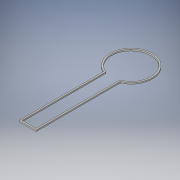
# Autodesk Inventor part: Arm Layer 2 Out
Saved by Autodesk Inventor 2016 (Build 200138000, 138)
## iProperties
Created: 2016-04-16
Part Number: Arm Layer 2 Out
Material: Generic
Document SubType Name: Modeling
Designer: rmarkowi
Density: 1 g/cm^3
Appearance: Default
Author: rmarkowi
Autodesk Inventor part; units mm, degrees
ref_plane "YZ Plane" through (0, 0, 0) normal (1, 0, 0) x (0, 1, 0)
ref_plane "XZ Plane" through (0, 0, 0) normal (0, 1, 0) x (-1, 0, 0)
ref_plane "XY Plane" through (0, 0, 0) normal (0, 0, 1) x (1, 0, 0)
sketch "Sketch1" plane through (0, 0, 0) normal (0, 1, 0) x (-1, 0, 0)
  line L0 (0, 0) -> (152.4, 0)
  line L1 (152.4, 0) -> (152.4, -762)
  line L2 (0, -762) -> (0, 0)
  line L3 (152.4, -762) -> (0, -762) construction
  arc A0 (0, -762) -> (152.4, -762) centre (76.2, -936.5961) ccw
  line L4 (152.4, -590.1365) -> (152.4, -762) construction
  arc A1 (12.7, -770.5221) -> (139.7, -770.5221) centre (76.2, -936.5961) ccw
  line L5 (12.7, -12.7) -> (139.7, -12.7)
  line L6 (139.7, -12.7) -> (139.7, -749.3)
  line L7 (12.7, -749.3) -> (12.7, -12.7)
  line L8 (12.7, -12.7) -> (139.7, -749.3) construction
  line L9 (139.7, -12.7) -> (12.7, -749.3) construction
  line L10 (12.7, -749.3) -> (12.7, -770.5221)
  line L11 (139.7, -749.3) -> (139.7, -770.5221)
  point P0 (76.2, -381)
  dimension "d0" = 762
  dimension "d1" = 381
  dimension "d2" = 355.6
  dimension "d3" = 762
  dimension "d4" = 127
  dimension "d5" = 736.6
  constraints: 24 end point, 4 point on circle, 3 parallel, 3 perpendicular, 2 centre point, 2 horizontal, 2 midpoint, 1 coincident, 1 collinear, 1 point on line
  measures "d0" distance of L0.end L1.end
  measures "d1" diameter of A0
  measures "d2" diameter of A1
  measures "d3" distance of L2.start L0.start
  measures "d4" distance of L6.end L7.start
  measures "d5" distance of L5.end L6.end
extrude "Extrusion1" add sketch "Sketch1" along normal blind 12.7
body "Solid1"
